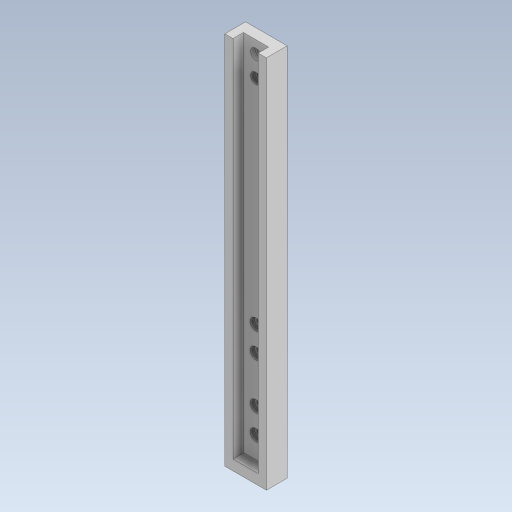
# Autodesk Inventor part: Tiang Lifter
Saved by Autodesk Inventor 2023.5 (Build 275446000, 446)
## iProperties
Created: 2025-09-06
Part Number: Tiang Lifter
Material: Generic
Document SubType Name: Modeling
Designer: Guntur
Density: 1 g/cm^3
Appearance: Default
Author: Guntur
## iProperties of the stored document Tiang Lifter_3DPrint.ipt
Created: 2025-09-06
Part Number: Tiang Lifter_3DPrint
Material: Generic
Document SubType Name: Modeling
Designer: Guntur
Density: 1 g/cm^3
Appearance: Default
Author: Guntur
Autodesk Inventor part; units mm, degrees
ref_plane "YZ Plane" through (0, 0, 0) normal (1, 0, 0) x (0, 1, 0)
ref_plane "XZ Plane" through (0, 0, 0) normal (0, 1, 0) x (-1, 0, 0)
ref_plane "XY Plane" through (0, 0, 0) normal (0, 0, 1) x (1, 0, 0)
sketch "Sketch1" plane through (0, 0, 0) normal (1, 0, 0) x (0, 1, 0)
  line L0 (75, 5) -> (-75, 5)
  line L1 (-75, 5) -> (-75, -5)
  line L2 (-75, -5) -> (75, -5)
  line L3 (75, -5) -> (75, 5)
  line L4 (75, 5) -> (-75, -5) construction
  line L5 (-75, 5) -> (75, -5) construction
  point P0 (0, 0)
  dimension "d0" = 150
  dimension "d1" = 10
  constraints: 12 end point, 2 midpoint, 2 parallel, 1 horizontal, 1 perpendicular
  measures "d0" distance of L2.end L1.end
  measures "d1" distance of L1.end L0.end
extrude "Extrusion1" add sketch "Sketch1" along normal blind 20
sketch "Sketch2" plane through (0, 75, 5) normal (0, 1, 0) x (1, 0, 0)
  line L0 (16.05, -5) -> (3.95, -5)
  line L1 (3.95, -5) -> (3.95, 5)
  line L2 (3.95, 5) -> (16.05, 5)
  line L3 (16.05, 5) -> (16.05, -5)
  line L4 (0, 0) -> (20, 0) projected
  line L5 (16.05, -5) -> (3.95, 5) construction
  line L6 (3.95, -5) -> (16.05, 5) construction
  point P0 (0, 5)
  point P1 (10, 0)
  point P2 (3.95, 0)
  point P3 (16.05, 0)
  dimension "d4" = 12.1
  constraints: 12 end point, 3 midpoint, 2 parallel, 1 horizontal, 1 perpendicular
  measures "d4" distance of L1.end L2.end
extrude "Extrusion2" cut sketch "Sketch2" against normal blind 145 contours L4 L1 L2 L3
sketch "Sketch3" plane through (3.95, 75, 0) normal (0, 0, 1) x (1, 0, 0)
  circle A0 centre (6.05, -134.5) radius 1.5
  line L0 (0, -145) -> (0, 0) projected
  line L1 (12.1, -145) -> (0, -145) projected
  circle A1 centre (6.05, -122.5) radius 1.5
  circle A2 centre (6.05, -122.5) radius 2.75
  circle A3 centre (6.05, -134.5) radius 2.75
  line L2 (1.5875, -111.5) -> (10.0422, -111.5)
  circle A4 centre (6.05, -88.5) radius 1.5
  circle A5 centre (6.05, -100.5) radius 1.5
  circle A6 centre (6.05, -100.5) radius 2.75
  circle A7 centre (6.05, -88.5) radius 2.75
  point P0 (-3.95, -75)
  point P1 (6.05, -145)
  dimension "d7" = 3
  dimension "d8" = 6.05
  dimension "d9" = 10.5
  dimension "d10" = 3
  dimension "d11" = 12
  dimension "d12" = 5.5
  dimension "d13" = 5.5
  dimension "d34" = 11
  constraints: 8 centre point, 4 coincident, 4 symmetric about line, 2 end point, 1 horizontal, 1 midpoint, 4 other
  measures "d7" diameter of A0
  measures "d8" distance from line of L0 A0.centre
  measures "d9" distance of point (6.05, -145) A0.centre
  measures "d10" diameter of A1
  measures "d11" distance of A0.centre A1.centre
  measures "d12" diameter of A2
  measures "d13" diameter of A3
  measures "d34" distance from line of A1.centre L2
extrude "Extrusion3" cut sketch "Sketch3" against normal blind 5 contours A0 | A1 | A4 | A5
extrude "Extrusion4" cut sketch "Sketch3" against normal blind 2
sketch "Sketch4" plane through (0, 75, 5) normal (0, 1, 0) x (1, 0, 0)
  line L0 (0, 0) -> (0, 10) projected
  line L1 (0, 0) -> (0, 10)
  line L2 (20, 0) -> (20, 10) projected
  line L3 (0, 10) -> (20, 10)
  line L4 (20, 10) -> (20, 0)
  line L5 (16.05, 5) -> (16.05, 0) projected
  line L6 (20, 0) -> (16.05, 0)
  line L7 (3.95, 5) -> (16.05, 5) projected
  line L8 (16.05, 0) -> (16.05, 5)
  line L9 (16.05, 5) -> (3.95, 5)
  line L10 (3.95, 0) -> (3.95, 5) projected
  line L11 (3.95, 5) -> (3.95, 0)
  line L12 (3.95, 0) -> (0, 0)
  point P0 (0, 5)
  constraints: 16 end point, 5 perpendicular, 3 collinear
extrude "Extrusion5" add sketch "Sketch4" along normal blind 30
sketch "Sketch6" plane through (3.95, -70, 0) normal (0, 0, 1) x (1, 0, 0)
  circle A0 centre (6.05, 169) radius 1.5
  circle A1 centre (6.05, 159) radius 1.5
  line L0 (0, 175) -> (12.1, 175) projected
  circle A2 centre (6.05, 169) radius 2.5
  circle A3 centre (6.05, 159) radius 2.5
  point P0 (-3.95, 70)
  point P1 (6.05, 175)
  dimension "d24" = 3
  dimension "d25" = 3
  dimension "d26" = 6
  dimension "d27" = 10
  dimension "d28" = 5
  dimension "d29" = 5
  constraints: 4 centre point, 2 coincident, 1 midpoint
  measures "d24" diameter of A0
  measures "d25" diameter of A1
  measures "d26" distance of point (6.05, 175) A0.centre
  measures "d27" distance of A0.centre A1.centre
  measures "d28" diameter of A2
  measures "d29" diameter of A3
extrude "Extrusion6" cut sketch "Sketch6" against normal blind 5 contours A0 | A1
extrude "Extrusion7" cut sketch "Sketch6" against normal blind 2 contours A1 | A2 | A3
body "Solid1"
